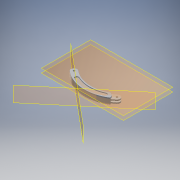
# Autodesk Inventor part: CurvedArm_test
Saved by Autodesk Inventor 2019 (Build 230136000, 136)
## iProperties
Created: 2018-06-20
Part Number: CurvedArm_test
Material: ABS Plastic
Document SubType Name: Modeling
Designer: car
Density: 1.06 g/cm^3
Appearance: Smooth - White
Mass: 21.8016 g
Surface Area: 95.9623 cm^2
Volume: 20.5675 cm^3
iToolsLastSavedTime: 02-07-2018 09:24:01
iToolsLastSavedBy: car
iToolsMass: 0,000
LastSavedDate: 02-07-2018
LastSavedTime: 09:24:01
LastSavedBy: CAR
Reserved: False
Title: =<Part number>
Author: car
Autodesk Inventor part; units mm, degrees
ref_plane "YZ Plane" through (0, 0, 0) normal (1, 0, 0) x (0, 1, 0)
ref_plane "XZ Plane" through (0, 0, 0) normal (0, 1, 0) x (-1, 0, 0)
sketch "Sketch1" plane through (0, 0, 0) normal (0, 0, 1) x (1, 0, 0)
  arc A0 (-51.423, 18.7164) -> (51.423, 18.7164) centre (0, 80) ccw construction
  line L0 (-51.423, 18.7164) -> (0, 80) construction
  line L1 (0, 80) -> (51.423, 18.7164) construction
  arc A1 (-46.6021, 24.4618) -> (-56.2439, 12.9711) centre (-51.423, 18.7164) ccw
  arc A2 (56.2439, 12.9711) -> (46.6021, 24.4618) centre (51.423, 18.7164) ccw
  arc A3 (-46.6021, 24.4618) -> (46.6021, 24.4618) centre (0, 80) ccw
  arc A4 (-56.2439, 12.9711) -> (56.2439, 12.9711) centre (0, 80) ccw
  line L2 (-51.423, 18.7164) -> (0, 80)
  line L3 (51.423, 18.7164) -> (0, 80)
  line L4 (0, 80) -> (-33.8095, 7.4954) construction
  line L5 (0, 80) -> (33.8095, 7.4954) construction
  arc A5 (-31.9077, 11.5738) -> (-35.7112, 3.417) centre (-33.8095, 7.4954) ccw
  arc A6 (35.7112, 3.417) -> (31.9077, 11.5738) centre (33.8095, 7.4954) ccw
  arc A7 (-31.9077, 11.5738) -> (31.9077, 11.5738) centre (0, 80) ccw
  arc A8 (-35.7112, 3.417) -> (35.7112, 3.417) centre (0, 80) ccw
  circle A9 centre (-51.423, 18.7164) radius 2
  circle A10 centre (51.423, 18.7164) radius 2
  point P0 (0, 0)
  point P1 (0, 0)
  dimension "Angel" = 80
  dimension "Radius" = 80
  dimension "d4" = 15
  dimension "d5" = 15
  dimension "d6" = 7.5
  dimension "d7" = 7.5
  dimension "d12" = 15
  dimension "d13" = 15
  dimension "d14" = 9
  dimension "d15" = 3
  dimension "d16" = 3
  dimension "d36" = 4
  dimension "d37" = 4
  constraints: 22 point on circle, 12 end point, 11 centre point, 6 coincident, 2 vertical alignment, 1 collinear, 1 equal radius, 1 horizontal alignment
  measures "Angel" angle of L1 L0
  measures "Radius" radius of A0
  measures "d4" diameter of A1
  measures "d5" diameter of A2
  measures "d6" radial gap between concentric circles of A0 A3
  measures "d7" radial gap between concentric circles of A0 A4
  measures "d12" angle of L1 L5
  measures "d13" angle of L0 L4
  measures "d14" diameter of A5
  measures "d15" radial gap between concentric circles of A3 A7
  measures "d16" radial gap between concentric circles of A4 A8
  measures "d36" diameter of A9
  measures "d37" diameter of A10
surface extrude "ExtrusionSrf1" sketch "Sketch1" along normal mid plane 30 shown yes curves L2 L3
ref_plane "Work Plane1" through (-51.423, 18.7164, 0) normal (-0.6427876, -0.7660444, 0) x (0, 0, 1)
ref_plane "Work Plane2" through (51.423, 18.7164, 0) normal (0.6427876, -0.7660444, 0) x (0, 0, -1)
extrude "Extrusion2" add sketch "Sketch1" along normal mid plane 15 contours A3 A2 A4 A1 | A7 A6 A8 A5
ref_plane "Work Plane3" through (0, 0, -5) normal (0, 0, 1) x (1, 0, 0)
ref_plane "Work Plane4" through (0, 0, 5) normal (0, 0, 1) x (1, 0, 0)
extrude "Extrusion3" cut sketch "Sketch1" along normal up to surface (2.5 mm away) from surface at 5 contours A7 A6 A8 A5
sketch "Sketch3" plane through (51.423, 18.7164, 0) normal (0.6427876, -0.7660444, 0) x (0, 0, -1)
  line L0 (-10.5, 0) -> (10.5, 0) projected
  line L1 (7.5, 7.5) -> (-7.5, 7.5) projected
  line L2 (1.5, 7.5) -> (-1.5, 7.5)
  line L3 (-1.5, 7.5) -> (-1.5, -8)
  line L4 (-1.5, -8) -> (1.5, -8)
  line L5 (1.5, -8) -> (1.5, 7.5)
  line L6 (-7.5, 0) -> (-7.5, -86.1707) projected
  line L7 (-4.5, 7.5) -> (-7.5, 7.5)
  line L8 (-7.5, 7.5) -> (-7.5, -8)
  line L9 (-7.5, -8) -> (-4.5, -8)
  line L10 (-4.5, -8) -> (-4.5, 7.5)
  line L11 (7.5, -86.1707) -> (7.5, 0) projected
  line L12 (4.5, 7.5) -> (7.5, 7.5)
  line L13 (7.5, 7.5) -> (7.5, -8)
  line L14 (7.5, -8) -> (4.5, -8)
  line L15 (4.5, -8) -> (4.5, 7.5)
  line L16 (4.5, -8) -> (1.5, -8)
  line L17 (-4.5, -8) -> (-1.5, -8)
  point P0 (0, -51.423)
  point P1 (-7.5, -86.1707)
  point P2 (0, -8)
  point P3 (0, 7.5)
  dimension "d23" = 8
  dimension "d24" = 3
  dimension "d25" = 3
  dimension "d26" = 3
  constraints: 28 end point, 8 equal length, 6 point on line, 3 horizontal, 3 midpoint, 3 perpendicular, 1 collinear, 1 vertical alignment
  measures "d23" distance between parallel lines of L14 L0
  measures "d24" distance between parallel lines of L3 L5
  measures "d25" distance between parallel lines of L15 L5
  measures "d26" distance between parallel lines of L10 L3
revolve "Revolution1" cut sketch "Sketch3" angle 225 mid plane about axis through (45.2947, 13.5741, 1.5) along (0, 0, -1) contours L8 L1 L10 L0 | L0 L10 L9 L6 | L3 L1 L5 L0 | L0 L5 L4 L3 | L15 L1 L13 L0 | L0 L11 L14 L15
sketch "Sketch5" plane through (-51.423, 18.7164, 0) normal (-0.6427876, -0.7660444, 0) x (0, 0, 1)
  line L0 (1.5, 7.5) -> (-1.5, 7.5)
  line L1 (-1.5, 7.5) -> (-1.5, -8)
  line L2 (-1.5, -8) -> (1.5, -8)
  line L3 (1.5, -8) -> (1.5, 7.5)
  line L4 (-4.5, 7.5) -> (-7.5, 7.5)
  line L5 (-7.5, 7.5) -> (-7.5, -8)
  line L6 (-7.5, -8) -> (-4.5, -8)
  line L7 (-4.5, -8) -> (-4.5, 7.5)
  line L8 (4.5, 7.5) -> (7.5, 7.5)
  line L9 (7.5, 7.5) -> (7.5, -8)
  line L10 (7.5, -8) -> (4.5, -8)
  line L11 (4.5, -8) -> (4.5, 7.5)
  line L12 (4.5, -8) -> (1.5, -8)
  line L13 (-4.5, -8) -> (-1.5, -8)
  line L14 (-7.5, 0) -> (-7.5, -83.6281) projected
  line L15 (7.5, -83.6281) -> (7.5, 0) projected
  line L16 (-10.5, 0) -> (10.5, 0) projected
  line L17 (0, 40.5) -> (0, -190.5) projected
  line L18 (4.5, 7.5) -> (1.5, 7.5)
  line L19 (-1.5, 7.5) -> (-4.5, 7.5)
  point P0 (0, -81.9152)
  point P1 (-7.5, -101.017)
  point P2 (7.5, -101.017)
  point P3 (0, -8)
  point P4 (0, 7.5)
  point P5 (-7.5, -83.6281)
  point P6 (7.5, -83.6281)
  dimension "d30" = 3
  dimension "d31" = 3
  dimension "d32" = 3
  dimension "d33" = 7.5
  dimension "d34" = 8
  constraints: 32 end point, 8 equal length, 5 collinear, 5 perpendicular, 3 horizontal, 2 midpoint, 2 point on line, 1 vertical alignment
  measures "d30" distance between parallel lines of L1 L3
  measures "d31" distance between parallel lines of L11 L3
  measures "d32" distance between parallel lines of L7 L1
  measures "d33" distance between parallel lines of L8 L16
  measures "d34" distance between parallel lines of L12 L16
revolve "Revolution2" cut sketch "Sketch5" angle 225 mid plane about axis through (-45.2947, 13.5741, 4.5) along (0, 0, -1) contours L18 L11 L16 L3 | L16 L11 L12 L3 | L1 L16 L7 L19 | L1 L13 L7 L16
mirror "Mirror1" about plane through (0, 0, 0) normal (0, 0, 1) of "Extrusion3"
fillet "Fillet1" radius 10 5 edges at (-45.2947, 13.5741, -3) (-45.2947, 13.5741, 3) (45.2947, 13.5741, 0) (45.2947, 13.5741, 6) (45.2947, 13.5741, -6)
fillet "Fillet2" radius 0.5 32 edges at (44.6635, 13.0445, 4.5) (47.0285, 8.075, 4.5) (39.4177, 16.6335, 4.5) (44.6635, 13.0445, -1.5) (47.0285, 8.075, -1.5) (39.4177, 16.6335, -1.5) (44.6635, 13.0445, 1.5) (47.0285, 8.075, 1.5) (39.4177, 16.6335, 1.5) (44.6635, 13.0445, -4.5) (47.0285, 8.075, -4.5) (39.4177, 16.6335, -4.5) (-44.6635, 13.0445, -4.5) (-47.0285, 8.075, -4.5) (-39.4177, 16.6335, -4.5) (-44.6635, 13.0445, -1.5) (-47.0285, 8.075, -1.5) (-39.4177, 16.6335, -1.5) (-44.6635, 13.0445, 4.5) (-47.0285, 8.075, 4.5) (-39.4177, 16.6335, 4.5) (-44.6635, 13.0445, 1.5) (-47.0285, 8.075, 1.5) (-39.4177, 16.6335, 1.5) (37.8878, 9.3972, -5) (0, -4.5, -5) (-37.8878, 9.3972, -5) (0, 4.5, -5) (37.8878, 9.3972, 5) (0, -4.5, 5) (-37.8878, 9.3972, 5) (0, 4.5, 5)
fillet "Fillet3" radius 0.2 50 edges at (37.3602, 17.8674, -4.6485) (37.2149, 17.7802, -6.25) (57.1683, 23.5374, -4.5) (52.1889, 9.7678, -4.5) (47.6387, 6.6051, -4.6531) (47.5169, 6.5262, -6.25) (42.2797, 21.1045, -4.5) (37.3602, 17.8674, 1.3515) (37.2149, 17.7802, 0) (37.3602, 17.8674, -1.3515) (42.2797, 21.1045, -1.5) (57.1683, 23.5374, -1.5) (52.1889, 9.7678, -1.5) (47.6387, 6.6051, -1.3469) (47.5169, 6.5262, 0) (47.6387, 6.6051, 1.3469) (52.1889, 9.7678, 1.5) (57.1683, 23.5374, 1.5) (42.2797, 21.1045, 1.5) (57.1683, 23.5374, 4.5) (52.1889, 9.7678, 4.5) (47.6387, 6.6051, 4.6531) (47.5169, 6.5262, 6.25) (37.3602, 17.8674, 4.6485) (37.2149, 17.7802, 6.25) (42.2797, 21.1045, 4.5) (-37.3602, 17.8674, -4.3515) (-37.2149, 17.7802, -3) (-37.3602, 17.8674, -1.6485) (-42.2797, 21.1045, -1.5) (-57.1683, 23.5374, -1.5) (-52.1889, 9.7678, -1.5) (-47.6387, 6.6051, -1.6531) (-47.5169, 6.5262, -3) (-47.6387, 6.6051, -4.3469) (-52.1889, 9.7678, -4.5) (-57.1683, 23.5374, -4.5) (-42.2797, 21.1045, -4.5) (-37.3602, 17.8674, 1.6485) (-37.2149, 17.7802, 3) (-37.3602, 17.8674, 4.3515) (-42.2797, 21.1045, 4.5) (-57.1683, 23.5374, 4.5) (-52.1889, 9.7678, 4.5) (-47.6387, 6.6051, 4.3469) (-47.5169, 6.5262, 3) (-47.6387, 6.6051, 1.6531) (-52.1889, 9.7678, 1.5) (-57.1683, 23.5374, 1.5) (-42.2797, 21.1045, 1.5)
fillet "Fillet4" radius 0.5 24 edges at (37.2158, 17.7512, -7.5) (39.4672, 16.6077, -7.5) (44.6635, 13.0445, -7.5) (47.0056, 8.1477, -7.5) (47.4684, 6.5436, -7.5) (-5.5006, -7.3269, -7.5) (-57.1683, 23.5374, -7.5) (-5.8167, 7.7337, -7.5) (-57.1683, 23.5374, 7.5) (-5.5006, -7.3269, 7.5) (47.4684, 6.5436, 7.5) (47.0056, 8.1477, 7.5) (44.6635, 13.0445, 7.5) (39.4672, 16.6077, 7.5) (37.2158, 17.7512, 7.5) (-5.8167, 7.7337, 7.5) (-37.8878, 9.3972, 7.5) (0, 4.5, 7.5) (37.8878, 9.3972, 7.5) (0, -4.5, 7.5) (37.8878, 9.3972, -7.5) (0, 4.5, -7.5) (-37.8878, 9.3972, -7.5) (0, -4.5, -7.5)
sketch "Sketch6" plane through (0, 0, -7.5) normal (0, 0, -1) x (-1, 0, 0)
  circle A0 centre (51.423, 18.7164) radius 2 projected
  circle A1 centre (51.423, 18.7164) radius 6
  point P0 (0, 0)
  dimension "d42" = 12
  constraints: 1 centre point, 1 coincident
  measures "d42" diameter of A1
extrude "Extrusion4" add sketch "Sketch6" along normal blind 2
sketch "Sketch7" plane through (-51.423, 18.7164, -9.5) normal (0, 0, -1) x (-1, 0, 0)
  circle A0 centre (0, 0) radius 2 projected
  circle A1 centre (0, 0) radius 6 projected
  line L0 (2.3671, 4.1) -> (4.7343, 0)
  line L1 (4.7343, 0) -> (2.3671, -4.1)
  line L2 (2.3671, -4.1) -> (-2.3671, -4.1)
  line L3 (-2.3671, -4.1) -> (-4.7343, 0)
  line L4 (-4.7343, 0) -> (-2.3671, 4.1)
  line L5 (-2.3671, 4.1) -> (2.3671, 4.1)
  point P0 (-51.423, -18.7164)
  dimension "d45" = 8.2
  constraints: 12 end point, 1 coincident, 13 other
  measures "d45" distance between parallel lines of L2 L5
extrude "Extrusion5" cut sketch "Sketch7" against normal blind 2 contours L0 L1 L2 L3 L4 L5
fillet "Fillet5" radius 0.2 2 edges at (-45.423, 18.7164, -7.5) (-45.423, 18.7164, -9.5)
chamfer "Chamfer1" distance 0.2 angle 45 10 edges at (-53.423, 18.7164, -7.5) (-53.423, 18.7164, -4.5) (-53.423, 18.7164, -1.5) (-53.423, 18.7164, 1.5) (-53.423, 18.7164, 4.5) (-53.423, 18.7164, 7.5) (49.423, 18.7164, 4.5) (49.423, 18.7164, 1.5) (49.423, 18.7164, -1.5) (49.423, 18.7164, -4.5)
equation "\"d13\" = d12"
body "Solid2"
body "Srf1"
